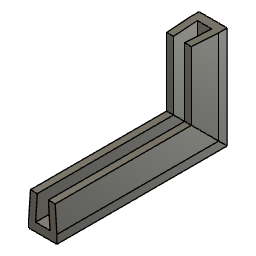
cover-edges-corner (Autodesk Fusion 360 design; units mm, degrees)
Autodesk Fusion 360 part; units mm, degrees
sketch "Sketch1" plane through (0, 0, 0) normal (0, 0, 1) x (1, 0, 0)
  line L0 (0, 7.5) -> (0, -2.5) construction
  line L1 (-4.125, 0) -> (4.125, 0) construction
  line L2 (-3.625, 7.5) -> (-4.125, 0)
  line L3 (-4.125, -2.5) -> (4.125, -2.5)
  line L4 (4.125, -2.5) -> (4.125, 0)
  line L5 (4.125, 0) -> (3.625, 7.5)
  line L6 (3.625, 7.5) -> (1.625, 7.5)
  line L7 (1.625, 7.5) -> (2.125, 0)
  line L8 (-2.125, 0) -> (-1.625, 7.5)
  line L9 (-1.625, 7.5) -> (-3.625, 7.5)
  line L10 (-2.125, 0) -> (2.125, 0)
  line L11 (-3.8098, 4.7284) -> (-1.8142, 4.5954) construction
  line L12 (-4.125, 0) -> (-4.125, -2.5)
  dimension "d7" = 7.5
  dimension "d8" = 8.25
  dimension "d9" = 4.25
  dimension "d10" = 3.25
  dimension "d12" = 2
  dimension "d13" = 2.5
  constraint vertical L0
  constraint perpendicular L0 L1
  constraint horizontal origin L1.end
  constraint vertical origin L0.start
  constraint symmetric L0 L1.start L1.end
  constraint perpendicular L4 L6
  constraint coincident L1 L7.end
  constraint coincident L1 L8.start
  constraint symmetric L0 L7.end L8.start
  constraint horizontal L9
  constraint horizontal L6
  constraint horizontal L6.end L8.end
  constraint symmetric L0 L6.end L8.end
  constraint horizontal L0.start L8.end
  constraint parallel L2 L8
  constraint parallel L5 L7
  constraint coincident L2 L11.start
  constraint perpendicular L8 L11
  constraint perpendicular L1 L12
  constraint horizontal L3
  constraint coincident L3.end L4.start
  constraint coincident L3 L0.end
  measures "d7" distance of origin L0.start
  measures "d8" distance of L1.start L1.end
  measures "d9" distance of L7.end L8.start
  measures "d10" distance of L6.end L8.end
  measures "d12" distance of L11.start L11.end
  measures "d13" distance of origin L0.end
extrude "Extrude1" add sketch "Sketch1" along normal blind 50 makes body 1
ref_plane "WorkPlane1" through (0, -2.5, 0) normal (0, -0.707107, 0.707107) x (1, 0, 0)
sketch "Sketch2" plane through (0, -2.5, 0) normal (0, -0.707107, 0.707107) x (1, 0, 0)
  line L0 (20, 20) -> (-20, 20)
  line L1 (-20, 20) -> (-20, -15)
  line L2 (-20, -15) -> (20, -15)
  line L3 (20, -15) -> (20, 20)
  constraint horizontal L0
  constraint vertical L1
  constraint horizontal L2
  constraint vertical L3
extrude "Extrude2" cut sketch "Sketch2" against normal through all bodies 1
extrude "Extrude3" add sketch "Sketch1" against normal blind 30 separate body makes body 2
move_body "Move1" bodies 2 to x (1, 0, 0) y (0, 0, 1) z (0, -1, 0) at (0, -2.5, 2.5)
extrude "Extrude4" cut sketch "Sketch2" along normal through all bodies 2
equation "thickness_back = 2.5 mm"
equation "thickness_sides = 2 mm"
equation "length_sides = 7.5 mm"
equation "width_normal = 4.25 mm"
equation "width_pinch = 3.25 mm"
equation "d7 = length_sides"
equation "d8 = width_normal + 2 * thickness_sides"
equation "d9 = width_normal"
equation "d10 = width_pinch"
equation "d12 = thickness_sides"
equation "d13 = thickness_back"
